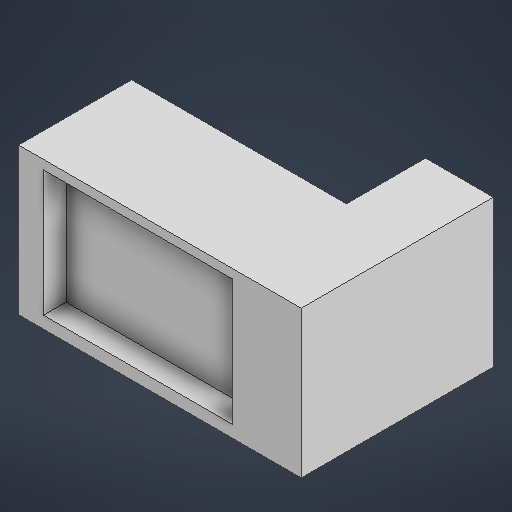
# Autodesk Inventor part: telo1
Saved by Autodesk Inventor 2026.2 (Build 302298000, 298)
## iProperties
Created: 2025-12-28
Part Number: telo1
Material: Všeobecné
Document SubType Name: Modeling
Designer: Vitek
Density: 1 g/cm^3
Appearance: Výchozí
Author: Vitek
Autodesk Inventor part; units mm, degrees
ref_plane "YZ Plane" through (0, 0, 0) normal (1, 0, 0) x (0, 1, 0)
ref_plane "XZ Plane" through (0, 0, 0) normal (0, 1, 0) x (-1, 0, 0)
ref_plane "XY Plane" through (0, 0, 0) normal (0, 0, 1) x (1, 0, 0)
sketch "Náčrt1" plane through (0, 0, 0) normal (0, 0, 1) x (1, 0, 0)
  line L0 (-62.5, 32.5) -> (62.5, 32.5)
  line L1 (62.5, 32.5) -> (62.5, -32.5)
  line L2 (62.5, -32.5) -> (-62.5, -32.5)
  line L3 (-62.5, -32.5) -> (-62.5, 32.5)
  line L4 (-87.5, 0) -> (87.5, 0) projected
  line L5 (0, 45.5) -> (0, -45.5) projected
  point P0 (0, 0)
  dimension "d0" = 125
  dimension "d1" = 65
  constraints: 8 end point, 2 parallel, 1 horizontal, 1 perpendicular, 2 other
  measures "d0" distance of L1.end L2.end
  measures "d1" distance of L0.end L1.end
extrude "Vysunutí1" add sketch "Náčrt1" along normal mid plane 50
sketch "Náčrt2" plane through (0, 0, -25) normal (0, 0, -1) x (-1, 0, 0)
  line L0 (-87.5, 0) -> (87.5, 0) projected
  circle A0 centre (15, 0) radius 27
  line L1 (0, -45.5) -> (0, 45.5) projected
  dimension "d18" = 54
  dimension "d19" = 15
  constraints: 1 centre point, 1 point on line
  measures "d18" diameter of A0
  measures "d19" distance from line of L1 A0.centre
extrude "Vysunutí2" cut sketch "Náčrt2" against normal blind 10
sketch "Náčrt3" plane through (0, 0, 25) normal (0, 0, 1) x (1, 0, 0)
  line L0 (32.02, 28.5) -> (-51.5, 28.5)
  line L1 (-51.5, 28.5) -> (-51.5, -27.18)
  line L2 (-51.5, -27.18) -> (32.02, -27.18)
  line L3 (32.02, -27.18) -> (32.02, 28.5)
  line L4 (-62.5, 32.5) -> (-62.5, -32.5) projected
  line L5 (62.5, 32.5) -> (-62.5, 32.5) projected
  point P0 (0, 0)
  dimension "d8" = 83.52
  dimension "d9" = 55.68
  dimension "d11" = 11
  dimension "d12" = 4
  constraints: 8 end point, 2 parallel, 1 horizontal, 1 perpendicular
  measures "d8" distance of L2.end L1.end
  measures "d9" distance of L1.end L0.end
  measures "d11" distance between parallel lines of L1 L4
  measures "d12" distance between parallel lines of L5 L0
extrude "Vysunutí3" cut sketch "Náčrt3" against normal blind 10
sketch "Náčrt4" plane through (0, 0, -25) normal (0, 0, -1) x (-1, 0, 0)
  line L0 (62.5, -32.5) -> (62.5, 32.5) projected
  line L1 (62.5, 32.5) -> (-62.5, 32.5) projected
  line L2 (-62.5, 32.5) -> (-62.5, -32.5) projected
  line L3 (-62.5, -32.5) -> (62.5, -32.5) projected
  line L4 (-62.5, 32.5) -> (-32.5, 32.5)
  line L5 (-32.5, 32.5) -> (-32.5, -33.9338)
  line L6 (-32.5, -33.9338) -> (-62.5, -33.9338)
  line L7 (-62.5, -33.9338) -> (-62.5, 32.5)
  point P0 (0, 0)
  point P1 (-32.5, -32.5)
  dimension "d15" = 30
  constraints: 8 end point, 2 parallel, 1 horizontal, 1 perpendicular
  measures "d15" distance of L5.end L6.end
extrude "Vysunutí4" add sketch "Náčrt4" along normal blind 35 contours L3 L2 L1 L5
